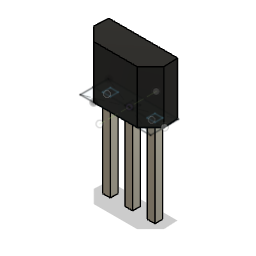
Hall_sensor_holder_tube_hall_holder (Autodesk Fusion 360 archive; units mm, degrees)
design "hall_sensor_49E_drawing"
Autodesk Fusion 360 part; units mm, degrees
sketch "Sketch1" plane through (0, 0, 0) normal (0, 1, 0) x (1, 0, 0)
  line L0 (2, -0.79) -> (-2, -0.79)
  line L1 (-2, -0.79) -> (-2, 0.79)
  line L2 (-2, 0.79) -> (2, 0.79)
  line L3 (2, 0.79) -> (2, -0.79)
  line L4 (2, -0.79) -> (-2, 0.79) construction
  line L5 (-2, -0.79) -> (2, 0.79) construction
  line L6 (2, 0) -> (2, -0.03)
  line L7 (2, -0.03) -> (-2, -0.03)
  line L8 (-2, -0.03) -> (-2, 0)
  line L9 (0, 1.5294) -> (0, -1.6799) construction
  line L10 (2, -0.03) -> (1.24, -0.79)
  line L11 (2, -0.03) -> (1.957, 0.79)
  line L12 (-2, -0.03) -> (-1.957, 0.79)
  line L13 (-2, -0.03) -> (-1.24, -0.79)
  line L14 (-0.22, -0.03) -> (0.22, -0.03)
  line L15 (0.22, -0.03) -> (0.22, 0.41)
  line L16 (0.22, 0.41) -> (-0.22, 0.41)
  line L17 (-0.22, 0.41) -> (-0.22, -0.03)
  line L18 (-1.49, -0.03) -> (-1.05, -0.03)
  line L19 (-1.05, 0.41) -> (-1.49, 0.41)
  line L20 (-1.05, -0.03) -> (-1.05, 0.41)
  line L21 (-1.49, 0.41) -> (-1.49, -0.03)
  line L22 (1.05, -0.03) -> (1.49, -0.03)
  line L23 (1.49, 0.41) -> (1.05, 0.41)
  line L24 (1.05, 0.41) -> (1.05, -0.03)
  line L25 (1.49, -0.03) -> (1.49, 0.41)
  point P0 (-1.27, 0)
  point P1 (-1.27, 0)
  point P2 (1.27, 0)
  point P3 (1.27, 0)
  dimension "d1" = 1.58
  dimension "d2" = 4
  dimension "d3" = 0.76
  dimension "d4" = 45
  dimension "d5" = 3
  dimension "d6" = 0.44
  dimension "d7" = 0.44
  dimension "d8" = 0.22
  dimension "d9" = 0.44
  dimension "d10" = 0.44
  dimension "d11" = 0.44
  dimension "d12" = 0.44
  constraint horizontal L0
  constraint perpendicular L0 L1
  constraint parallel L0 L2
  constraint parallel L1 L3
  constraint coincident L4 origin
  constraint coincident L5 origin
  constraint vertical L6
  constraint horizontal L7
  constraint vertical L8
  constraint coincident L3 L6.end
  constraint midpoint L1 L8.end
  constraint perpendicular L2 L9
  constraint coincident L0 L10.end
  constraint coincident L2 L11.end
  constraint symmetric L6.end L9 L7.end
  constraint symmetric L9 L10.end L13.end
  constraint symmetric L9 L11.end L12.end
  constraint horizontal L14
  constraint vertical L15
  constraint horizontal L16
  constraint vertical L17
  constraint coincident L7 L14.start
  constraint coincident P1 P0
  constraint horizontal L18
  constraint vertical L20
  constraint horizontal L19
  constraint vertical L21
  constraint coincident P3 P2
  constraint horizontal L22
  constraint vertical L25
  constraint horizontal L23
  constraint vertical L24
  measures "d1" distance of L0.end L1.end
  measures "d2" distance of L1.end L2.end
  measures "d3" distance of L0 L7
  measures "d4" angle of L0 L10
  measures "d5" angle of L3 L11
  measures "d6" distance of L15.end L16.end
  measures "d7" distance of L14.end L15.end
  measures "d8" distance of L9 L15
  measures "d9" distance of L19.start L19.end
  measures "d10" distance of L18.end L19.start
  measures "d11" distance of L23.start L23.end
  measures "d12" distance of L22.end L23.start
extrude "Extrude1" add sketch "Sketch1" along normal blind 3 contours L0 L7 L10 L13 L14 L18 L22 | L1 L2 L3 L6 L7 L8 L11 L12 L15 L16 L17 L19 L20 L21 L23 L24 L25 | L7 L22 L23 L24 L25 | L7 L18 L19 L20 L21 | L7 L14 L15 L16 L17 makes body 1
extrude "Extrude2" add sketch "Sketch1" against normal blind 5 contours L7 L22 L23 L24 L25 | L7 L18 L19 L20 L21 | L7 L14 L15 L16 L17 bodies 1
split "Split1" by plane through (0, 0, 0) normal (0, -1, 0) bodies 1 makes body 2 at (0.22, -1.6667, -0.1167) makes body 3 at (-1.49, -1.6667, -0.2633) makes body 4 at (1.49, -1.6667, -0.1167)
